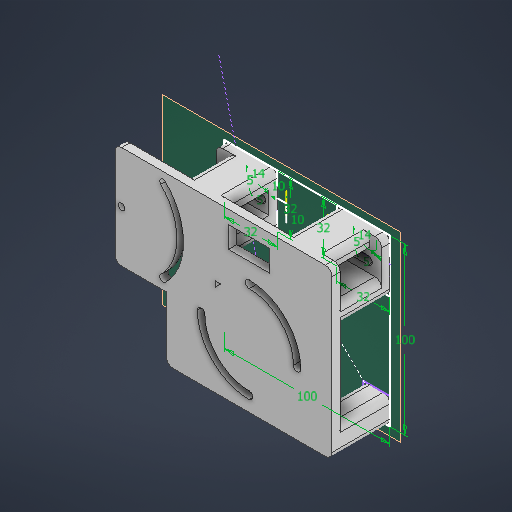
# Autodesk Inventor part: suporte_imu_lidar
Saved by Autodesk Inventor 2026.1 (Build 301233000, 233)
## iProperties
Created: 2026-03-31
Part Number: suporte_imu_lidar
Material: Generic
Document SubType Name: Modeling
Designer: fheli
Density: 1 g/cm^3
Appearance: Default
Author: fheli
Autodesk Inventor part; units mm, degrees
ref_plane "YZ Plane" through (0, 0, 0) normal (1, 0, 0) x (0, 1, 0)
ref_plane "XZ Plane" through (0, 0, 0) normal (0, 1, 0) x (-1, 0, 0)
ref_plane "XY Plane" through (0, 0, 0) normal (0, 0, 1) x (1, 0, 0)
sketch "Sketch1" plane through (0, 0, 0) normal (0, 0, 1) x (1, 0, 0)
  point P0 (0, 0)
sketch "Sketch2" plane through (0, 0, 0) normal (0, 0, 1) x (1, 0, 0)
  line L0 (-50, -50) -> (50, -50)
  line L1 (50, -50) -> (50, 50)
  line L2 (50, 50) -> (-50, 50)
  line L3 (0, 42) -> (12.5, 42)
  line L4 (12.5, 42) -> (12.5, 29)
  line L5 (12.5, 29) -> (-12.5, 29)
  line L6 (-12.5, 29) -> (-12.5, 42)
  line L7 (-12.5, 42) -> (0, 42)
  circle A0 centre (0, -12) radius 38
  line L8 (-19, 31) -> (-19, 20.909)
  line L9 (-50, 50) -> (-50, 31)
  line L10 (-50, -31) -> (-50, -50)
  line L11 (20.5, 8.5) -> (20.5, -32.5)
  line L12 (20.5, -32.5) -> (-20.5, -32.5)
  line L13 (-20.5, 8.5) -> (20.5, -32.5) construction
  line L14 (20.5, 8.5) -> (-20.5, -32.5) construction
  line L15 (0, 16.9914) -> (0, -40.9914)
  line L16 (28.9914, -12) -> (-28.9914, -12)
  arc A1 (0, 19.2414) -> (0, 14.7414) centre (0, 16.9914) ccw
  arc A2 (26.7414, -12) -> (31.2414, -12) centre (28.9914, -12) ccw
  arc A3 (0, -43.2414) -> (0, -38.7414) centre (0, -40.9914) ccw
  arc A4 (-26.7414, -12) -> (-31.2414, -12) centre (-28.9914, -12) ccw
  arc A5 (-17.1712, 8.5) -> (-20.5, 5.1712) centre (0, -12) ccw
  arc A6 (-31.2414, -12) -> (0, -43.2414) centre (0, -12) ccw
  arc A7 (31.2414, -12) -> (0, 19.2414) centre (0, -12) ccw
  arc A8 (-26.7414, -12) -> (0, -38.7414) centre (0, -12) ccw
  arc A9 (17.1712, -32.5) -> (20.5, -29.1712) centre (0, -12) ccw
  arc A10 (26.7414, -12) -> (0, 14.7414) centre (0, -12) ccw
  line L17 (-20.5, -32.5) -> (-20.5, -12)
  line L18 (-20.5, 5.1712) -> (-20.5, 8.5)
  line L19 (-20.5, 8.5) -> (-17.1712, 8.5)
  line L20 (0, 8.5) -> (20.5, 8.5)
  line L21 (-50, 31) -> (-50, -31)
  line L22 (-50, 50) -> (-81, 50)
  line L23 (-81, 50) -> (-81, 19)
  line L24 (-81, 19) -> (-81, -12)
  line L25 (-81, -12) -> (-50, -12)
  circle A11 centre (-77, 19) radius 2
  arc A12 (-50.5858, 45.4142) -> (-53.4142, 42.5858) centre (-52, 44) ccw
  arc A13 (-53.4142, -4.5858) -> (-50.5858, -7.4142) centre (-52, -6) ccw
  arc A14 (-53.4142, -4.5858) -> (-53.4142, 42.5858) centre (-77, 19) ccw
  arc A15 (-50.5858, -7.4142) -> (-50.5858, 45.4142) centre (-77, 19) ccw
  dimension "d15" = 76
  dimension "d0" = 100
  dimension "d1" = 100
  dimension "d4" = 13
  dimension "d5" = 25
  dimension "d6" = 13
  dimension "d25" = 41
  dimension "d26" = 41
  dimension "d29" = 4.5
  dimension "d30" = 4.5
  dimension "d31" = 4.5
  dimension "d32" = 4.5
  dimension "d35" = 31
  dimension "d36" = 31
  dimension "d37" = 31
  dimension "d38" = 4
  dimension "d43" = 4
  dimension "d44" = 4
  constraints: 52 end point, 28 point on circle, 15 centre point, 8 perpendicular, 7 coincident, 6 point on line, 5 horizontal, 5 parallel, 5 vertical, 2 midpoint, 3 other
  measures "d0" distance of L2.end L1.end
  measures "d1" distance of L1.end L0.end
  measures "d4" distance of L3.end L4.end
  measures "d5" distance of L4.end L5.end
  measures "d6" distance of L5.end L6.end
  measures "d25" distance of L11.end L12.end
  measures "d26" distance of L11.start L11.end
  measures "d29" diameter of A1
  measures "d30" diameter of A2
  measures "d31" diameter of A3
  measures "d32" diameter of A4
  measures "d35" distance of L2.end L22.end
  measures "d36" distance of L22.end L23.end
  measures "d37" distance of L23.end L24.end
  measures "d38" diameter of A11
  measures "d43" diameter of A12
  measures "d44" diameter of A13
sketch "Sketch3" plane through (0, 0, 0) normal (0, 0, 1) x (1, 0, 0)
  point P0 (0, 0)
sketch "Sketch4" plane through (0, 0, 0) normal (0, 0, 1) x (1, 0, 0)
  point P0 (0, 0)
extrude "Extrusion1" add sketch "Sketch2" along normal blind 5 contours A0 | L10 L21 A15 L9 L2 L1 L0 | L25 L24 L23 L22 L9 A15 A12 A14 L21 A13 | L21 L9 A14 | A9 L12 L15 L16 L11 | L11 L12 A9 | L16 L15 L20 A10 L11 | L11 A10 L16 | L15 L12 A8 L17 L16 | L15 A8 L12 | L20 L15 A10 | L17 A8 L16
fillet "Fillet1" radius 4 1 edges at (50, -50, 2.5)
fillet "Fillet2" radius 4 1 edges at (50, 50, 2.5)
fillet "Fillet3" radius 4 1 edges at (-81, 50, 2.5)
fillet "Fillet4" radius 4 1 edges at (-81, -12, 2.5)
fillet "Fillet5" radius 4 1 edges at (-50, -50, 2.5)
ref_plane "Work Plane1" through (0, 0, -30) normal (0, 0, -1) x (-1, 0, 0)
sketch "Sketch5" plane through (0, 0, -30) normal (0, 0, -1) x (-1, 0, 0)
  line L0 (50, 50) -> (-50, 50)
  line L1 (-50, 50) -> (-50, -50)
  line L2 (-50, -50) -> (50, -50)
  line L3 (50, -50) -> (50, 50)
  line L4 (50, 50) -> (-50, -50) construction
  line L5 (-50, 50) -> (50, -50) construction
  line L6 (-50, 50) -> (-18, 50)
  line L7 (-18, 50) -> (-18, 18)
  line L8 (-18, 18) -> (-50, 18)
  line L9 (-50, 18) -> (-50, 50)
  line L10 (50, 50) -> (18, 50)
  line L11 (18, 50) -> (18, 18)
  line L12 (18, 18) -> (50, 18)
  line L13 (50, 18) -> (50, 50)
  arc A0 (-41.7887, 38) -> (-41.7887, 33) centre (-41.7887, 35.5) ccw
  line L14 (-41.7887, 38) -> (-27.7887, 38)
  arc A1 (-27.7887, 33) -> (-27.7887, 38) centre (-27.7887, 35.5) ccw
  line L15 (-27.7887, 33) -> (-41.7887, 33)
  line L16 (53.501, 93.553) -> (26.3897, -19.2628) construction
  line L17 (-41.7887, 35.5) -> (-31.7887, 35.5) construction
  line L18 (-12.5, 42) -> (-12.5, 29) projected
  line L19 (-12.5, 35.5) -> (-50, 35.5)
  line L20 (12.5, 29) -> (12.5, 42) projected
  line L21 (12.5, 35.5) -> (12.5, 25.5)
  line L22 (12.5, 35.5) -> (22.5, 35.5)
  arc A2 (22.5, 38) -> (22.5, 33) centre (22.5, 35.5) ccw
  line L23 (22.5, 38) -> (36.5, 38)
  arc A3 (36.5, 33) -> (36.5, 38) centre (36.5, 35.5) ccw
  line L24 (36.5, 33) -> (22.5, 33)
  line L25 (22.5, 35.5) -> (32.5, 35.5) construction
  line L26 (18, 50) -> (42, 50)
  line L27 (42, 50) -> (42, 42)
  line L28 (42, 42) -> (18, 42)
  line L29 (18, 42) -> (18, 50)
  line L30 (18, 18) -> (37.9879, 18)
  line L31 (37.9879, 18) -> (37.9879, 29)
  line L32 (37.9879, 29) -> (18, 29)
  line L33 (18, 29) -> (18, 18)
  line L34 (-18, 50) -> (-42.975, 50)
  line L35 (-42.975, 50) -> (-42.975, 42.975)
  line L36 (-42.975, 42.975) -> (-18, 42.975)
  line L37 (-18, 42.975) -> (-18, 50)
  line L38 (-18, 18) -> (-50, 18)
  line L39 (-50, 18) -> (-50, 29)
  line L40 (-50, 29) -> (-18, 29)
  line L41 (-18, 29) -> (-18, 18)
  line L42 (-50, -50) -> (-34, -50)
  line L43 (-34, -50) -> (-34, -34)
  line L44 (-34, -34) -> (-50, -34)
  line L45 (-50, -34) -> (-50, -50)
  line L46 (50, -50) -> (34, -50)
  line L47 (34, -50) -> (34, -34)
  line L48 (34, -34) -> (50, -34)
  line L49 (50, -34) -> (50, -50)
  point P0 (0, 0)
  point P1 (-42.975, 44.7393)
  point P2 (39.9453, 37.1451)
  point P3 (-49.2669, 35.5)
  dimension "d53" = 100
  dimension "d54" = 100
  dimension "d55" = 32
  dimension "d56" = 32
  dimension "d57" = 32
  dimension "d58" = 32
  dimension "d59" = 5
  dimension "d60" = 14
  dimension "d62" = 5
  dimension "d71" = 10
  dimension "d72" = 10
  dimension "d73" = 5
  dimension "d74" = 14
  dimension "d75" = 5
  constraints: 96 end point, 18 parallel, 14 horizontal, 10 point on line, 9 perpendicular, 8 point on circle, 6 tangent, 5 midpoint, 4 centre point, 1 collinear
  measures "d53" distance of L2.end L1.end
  measures "d54" distance of L1.end L0.end
  measures "d55" distance of L7.end L8.end
  measures "d56" distance of L6.end L7.end
  measures "d57" distance of L12.end L11.end
  measures "d58" distance of L11.end L10.end
  measures "d59" diameter of A0
  measures "d60" distance of L14.start L14.end
  measures "d62" diameter of A1
  measures "d71" distance of L21.start L21.end
  measures "d72" distance of L21.start L22.end
  measures "d73" diameter of A2
  measures "d74" distance of L23.start L23.end
  measures "d75" diameter of A3
extrude "Extrusion2" add sketch "Sketch5" against normal blind 32.225 contours L27 L28 L11 L0 | L12 L11 L32 L31
extrude "Extrusion3" add sketch "Sketch5" against normal blind 5 contours L3 L12 L31 L32 L11 L28 L27 L0
extrude "Extrusion4" add sketch "Sketch5" against normal blind 33.575 contours L7 L36 L35 L0 | L7 L8 L1 L40
extrude "Extrusion5" add sketch "Sketch5" against normal blind 5 contours L35 L36 L7 L19 A1 L14 A0 L1 L0 | L7 L40 L1 L19 A0 L15 A1
fillet "Fillet6" radius 4 1 edges at (50, 50, -27.5)
fillet "Fillet7" radius 4 1 edges at (-50, 50, -27.5)
fillet "Fillet8" radius 4 1 edges at (-18, 50, -15)
fillet "Fillet9" radius 4 1 edges at (18, 50, -15)
fillet "Fillet10" radius 4 1 edges at (18, 18, -15)
fillet "Fillet11" radius 4 1 edges at (-18, 18, -15)
fillet "Fillet12" radius 4 1 edges at (-50, 18, -27.5)
fillet "Fillet13" radius 4 1 edges at (50, 18, -15)
fillet "Fillet14" radius 4 1 edges at (-42, 50, -12.5)
fillet "Fillet15" radius 4 1 edges at (-37.9879, 18, -12.5)
fillet "Fillet16" radius 4 1 edges at (42.975, 50, -12.5)
fillet "Fillet17" radius 4 1 edges at (50, 29, -12.5)
extrude "Extrusion6" add sketch "Sketch5" against normal blind 33.575 contours L3 L2 L47 L48 | L2 L1 L44 L43
fillet "Fillet18" radius 4 1 edges at (-50, -50, -13.2125)
fillet "Fillet19" radius 4 1 edges at (34, -50, -15)
fillet "Fillet20" radius 4 1 edges at (50, -50, -13.2125)
fillet "Fillet21" radius 4 1 edges at (50, -34, -15)
fillet "Fillet22" radius 4 4 edges at (-34, -50, -15) (-34, -34, -15) (-50, -34, -15) (34, -34, -15)
body "Solid1"
